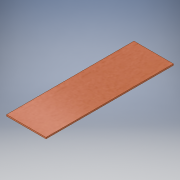
# Autodesk Inventor part: bett_V2_deckplatte_klappe
Saved by Autodesk Inventor 2018 (Build 220112000, 112)
## iProperties
Created: 2020-03-29
Part Number: bett_V2_deckplatte_klappe
Material: Holz (Walnuss)
Document SubType Name: Modeling
Designer: wepet
Density: 0.55 g/cm^3
Appearance: Walnuss - natur - poliert
Author: wepet
Autodesk Inventor part; units mm, degrees
ref_plane "YZ Plane" through (0, 0, 0) normal (1, 0, 0) x (0, 1, 0)
ref_plane "XZ Plane" through (0, 0, 0) normal (0, 1, 0) x (-1, 0, 0)
ref_plane "XY Plane" through (0, 0, 0) normal (0, 0, 1) x (1, 0, 0)
sketch "Skizze1" plane through (0, 0, 0) normal (0, 0, 1) x (1, 0, 0)
  line L0 (0, 0) -> (34, 0)
  line L1 (34, 0) -> (34, 110)
  line L2 (34, 110) -> (0, 110)
  line L3 (0, 110) -> (0, 91.5)
  line L4 (0, 86.5) -> (0, 91.5)
  line L5 (0, 18.5) -> (0, 23.5)
  line L6 (0, 23.5) -> (0, 18.5) construction
  line L7 (0, 18.5) -> (0, 0)
  line L8 (0, 86.5) -> (0, 23.5)
  line L9 (0, 91.5) -> (0, 86.5) construction
  dimension "d0" = 34
  dimension "d1" = 110
  constraints: 20 end point, 6 parallel, 1 horizontal, 1 perpendicular
  measures "d0" distance of L2.end L1.end
  measures "d1" distance of L1.end L0.end
extrude "Extrusion1" add sketch "Skizze1" along normal blind 1.2
